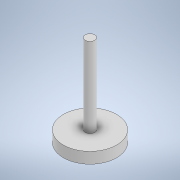
# Autodesk Inventor part: Millifluidic Board Assembly support
Saved by Autodesk Inventor 2021 (Build 250183000, 183)
## iProperties
Created: 2021-01-25
Part Number: Millifluidic Board Assembly support
Material: Generic
Document SubType Name: Modeling
Designer: natha
Density: 1 g/cm^3
Appearance: Default
Author: natha
Autodesk Inventor part; units mm, degrees
ref_plane "YZ Plane" through (0, 0, 0) normal (1, 0, 0) x (0, 1, 0)
ref_plane "XZ Plane" through (0, 0, 0) normal (0, 1, 0) x (-1, 0, 0)
ref_plane "XY Plane" through (0, 0, 0) normal (0, 0, 1) x (1, 0, 0)
sketch "Sketch2" plane through (0, 0, 0) normal (1, 0, 0) x (0, 1, 0)
  line L0 (0, 14.4) -> (0, -2.4) construction
  line L1 (5, 12) -> (0, 12)
  line L2 (0, 12) -> (0, 0)
  line L3 (0, 0) -> (5, 0)
  line L4 (5, 2.15) -> (5, 12)
  line L5 (5, 0) -> (41, 0)
  line L6 (41, 0) -> (41, 2.15)
  line L7 (41, 2.15) -> (5, 2.15)
  dimension "d0" = 12
  dimension "d1" = 2.15
  dimension "d2" = 5
  dimension "d3" = 36
  constraints: 14 end point, 3 parallel, 2 horizontal, 2 perpendicular
  measures "d0" distance between parallel lines of L3 L1
  measures "d1" distance between parallel lines of L5 L7
  measures "d2" distance between parallel lines of L4 L0
  measures "d3" distance between parallel lines of L4 L6
revolve "Revolution1" add sketch "Sketch2" angle 360 about axis through (0, 5, 0) along (0, 1, 0)
body "Solid1"
